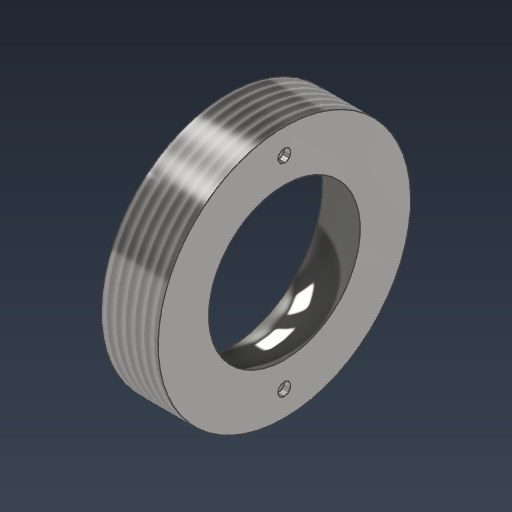
# Autodesk Inventor part: MCEN4000:T6
Saved by Autodesk Inventor 2021 (Build 250183000, 183)
## iProperties
Created: 2020-10-18
Part Number: MCEN4000:T6
Material: STEEL, AISI 1040
Document SubType Name: Modeling
Designer: Eugene Tang
Mass: 44.7853 g
Surface Area: 33.458 cm^2
Volume: 5.70513 cm^3
Density: 7.85 g/cm^3
Appearance: Steel - Polished
Description: TIE ROD OUTER CUP CAP
Author: Eugene Tang
Autodesk Inventor part; units mm, degrees
ref_plane "YZ Plane" through (0, 0, 0) normal (1, 0, 0) x (0, 1, 0)
ref_plane "XZ Plane" through (0, 0, 0) normal (0, 1, 0) x (-1, 0, 0)
ref_plane "XY Plane" through (0, 0, 0) normal (0, 0, 1) x (1, 0, 0)
ref_plane "Work Plane1" through (0, 0, 0) normal (0, 0, 1) x (1, 0, 0)
sketch "Sketch1" plane through (0, 0, 0) normal (0, 0, 1) x (1, 0, 0)
  line L0 (-8.678, -58.5397) -> (-8.678, 43.8978) construction
  line L1 (1.322, -54.9064) -> (1.322, 43.8978) construction
  circle A0 centre (-8.678, 43.8978) radius 15 construction
  line L2 (-8.678, 23.8978) -> (1.322, 23.8978) construction
  line L3 (0.322, 23.8978) -> (0.322, 31.8978)
  line L4 (-8.678, 28.8978) -> (-8.678, 23.8978)
  line L5 (-8.678, 23.8978) -> (0.322, 23.8978)
  arc A1 (-8.678, 28.8978) -> (0.322, 31.8978) centre (-8.678, 43.8978) ccw
  line L6 (-8.678, 43.8978) -> (1.322, 43.8978) construction
  point P0 (0, 0)
  dimension "d0" = 1
  constraints: 10 end point, 4 point on circle, 2 collinear, 2 horizontal, 1 centre point, 1 concentric, 1 point on line, 1 vertical, 2 other
  measures "d0" distance between parallel lines of L1 L3
revolve "Revolution1" add sketch "Sketch1" angle 360 about axis through (-8.678, 43.8978, 0) along (1, 0, 0)
thread "Thread2" size "M40x1.5" class "6g" standard "ISO Metric profile" length 9
sketch "Sketch9" plane through (0.322, 43.8978, 0) normal (1, 0, 0) x (0, 0, -1)
  circle A0 centre (0, 0) radius 12 construction
  circle A1 centre (0, 0) radius 20 construction
  circle A2 centre (0, 0) radius 16 construction
  line L0 (0, -56.6773) -> (0, 32.7796) construction
  circle A3 centre (0, -16) radius 1
  circle A4 centre (0, 16) radius 1
  point P0 (0, -43.8978)
  dimension "d49" = 4
  dimension "d50" = 8
  dimension "d51" = 2
  dimension "d52" = 2
  constraints: 3 centre point, 2 point on circle, 2 point on line, 1 coincident
  measures "d49" radial gap between concentric circles of A2 A0
  measures "d50" radial gap between concentric circles of A1 A0
  measures "d51" diameter of A4
  measures "d52" diameter of A3
extrude "Extrusion2" cut sketch "Sketch9" against normal blind 1
equation "\"d49\" = 0.5 * d50"
equation "\"d52\" = d51"
equation "\"d11\" = 55deg"
equation "\"Sketch2_Pitch\" = 1.5"
equation "\"d32\" = 55deg"
equation "\"Sketch5_Pitch\" = 1.5"
body "Solid1"
